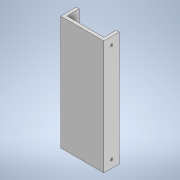
# Autodesk Inventor part: board-1-new
Saved by Autodesk Inventor 2020 (Build 240168000, 168)
## iProperties
Created: 2020-12-14
Part Number: board-1-new
Material: Типовые
Document SubType Name: Modeling
Designer: Alkhimov
Density: 1 g/cm^3
Appearance: По умолчанию
Author: Alkhimov
Autodesk Inventor part; units mm, degrees
ref_plane "YZ Plane" through (0, 0, 0) normal (1, 0, 0) x (0, 1, 0)
ref_plane "XZ Plane" through (0, 0, 0) normal (0, 1, 0) x (-1, 0, 0)
ref_plane "XY Plane" through (0, 0, 0) normal (0, 0, 1) x (1, 0, 0)
sketch "Эскиз1" plane through (0, 0, 0) normal (0, 1, 0) x (-1, 0, 0)
  line L0 (14, -5) -> (-14, -5)
  line L1 (-14, -5) -> (-14, 5)
  line L2 (-14, 5) -> (14, 5)
  line L3 (14, 5) -> (14, -5)
  line L4 (-14, -5) -> (14, 5) construction
  line L5 (14, -5) -> (-14, 5) construction
  line L6 (-12, -3) -> (12, -3)
  line L7 (12, -3) -> (12, 3)
  line L8 (12, 3) -> (-12, 3)
  line L9 (-12, 3) -> (-12, -3)
  point P0 (0, 0)
  point P1 (0, 0)
  dimension "d0" = 28
  dimension "d1" = 10
  dimension "d2" = 2
  constraints: 20 end point, 4 parallel, 2 perpendicular, 1 coincident, 1 horizontal, 1 midpoint, 3 other
  measures "d0" distance of L0.start L0.end
  measures "d1" distance of L0.end L1.end
  measures "d2" distance between parallel lines of L0 L6
extrude "Выдавливание1" add sketch "Эскиз1" along normal blind 74.2
sketch "Эскиз3" plane through (14, 0, -5) normal (0, 0, -1) x (-1, 0, 0)
  line L0 (0, 0) -> (0, 74.2) projected
  line L1 (28, 0) -> (28, 74.2) projected
  line L2 (28, 0) -> (28, 74.2) projected
  line L3 (0, 0) -> (0, 74.2) projected
  line L4 (0, 74.2) -> (28, 74.2) projected
  arc A0 (2, 64.2) -> (26, 64.2) centre (14, 64.2) ccw
  line L5 (26, 0) -> (26, 74.2) projected
  line L6 (2, 0) -> (2, 74.2) projected
  line L7 (26, 0) -> (26, 74.2) projected
  line L8 (26, 64.2) -> (26, 74.2)
  line L9 (26, 74.2) -> (2, 74.2)
  line L10 (2, 64.2) -> (2, 74.2)
  point P0 (14, 0)
  dimension "d10" = 10
  constraints: 6 end point, 3 tangent, 2 collinear, 2 point on circle, 2 point on line, 1 centre point, 1 perpendicular
  measures "d10" distance from line of L4 A0.centre
extrude "Выдавливание3" cut sketch "Эскиз3" against normal up to surface (2 mm away)
sketch "Эскиз2" plane through (14, 0, 5) normal (1, 0, 0) x (0, 0, -1)
  line L0 (0, 74.2) -> (10, 74.2) construction
  line L1 (10, 74.2) -> (0, 64.2) construction
  line L2 (0, 0) -> (0, 74.2) construction
  line L3 (0, 74.2) -> (10, 64.2) construction
  line L4 (10, 0) -> (10, 74.2) construction
  line L5 (10, 0) -> (0, 10) construction
  line L6 (0, 0) -> (10, 10) construction
  circle A0 centre (5, 69.2) radius 0.5
  circle A1 centre (5, 5) radius 0.5
  point P0 (5, 0)
  dimension "d5" = 1
  dimension "d6" = 1
  constraints: 8 end point, 4 perpendicular, 4 point on line, 2 centre point, 2 midpoint
  measures "d5" diameter of A0
  measures "d6" diameter of A1
hole "Отверстие1" at (14, 69.2, 0) at (14, 5, 0) direction (-1, 0, 0) diameter 1 depth 2 countersink diameter 1.5 countersink angle 90
mirror "Зеркальное отражение1" about plane through (0, 0, 0) normal (1, 0, 0) of "Отверстие1"
